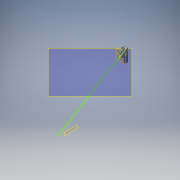
# Autodesk Inventor part: BracerBedMountpoint
Saved by Autodesk Inventor 2016 (Build 200138000, 138)
## iProperties
Created: 2016-05-27
Part Number: BracerBedMountpoint
Material: Generic
Document SubType Name: Modeling
Designer: Scott
Density: 1 g/cm^3
Appearance: Default
Author: Scott
Autodesk Inventor part; units mm, degrees
ref_plane "YZ Plane" through (0, 0, 0) normal (1, 0, 0) x (0, 1, 0)
ref_plane "Work Plane1" through (0, 0, 0) normal (0, 0, 1) x (1, 0, 0)
sketch "Sketch1" plane through (0, 0, 0) normal (0, 0, 1) x (1, 0, 0)
  circle A0 centre (-48.331, 27.8537) radius 2.5 projected
  circle A1 centre (30.6843, -32.9463) radius 2.5 projected
  circle A2 centre (30.6843, -1.1963) radius 2.5 projected
  circle A3 centre (-29.281, 27.8537) radius 2.5 projected
  line L0 (34.412, 17.8537) -> (34.412, 37.8537) projected
  line L1 (34.412, 17.8537) -> (-19.563, 17.8537) projected
  line L2 (-19.563, 37.8537) -> (-19.563, 17.8537) projected
  line L3 (-19.563, 37.8537) -> (-61.031, 37.8537) projected
  line L4 (-61.031, 37.8537) -> (-61.031, 17.8537) projected
  line L5 (-61.031, 17.8537) -> (20.7996, -58.3463) projected
  line L6 (20.7996, -58.3463) -> (40.569, -58.3463) projected
  line L7 (40.569, -58.3463) -> (40.569, 37.8537) projected
  line L8 (40.569, 37.8537) -> (34.412, 37.8537) projected
  line L9 (20.7996, 17.8537) -> (20.7996, -58.3463)
  line L10 (20.7996, 17.8537) -> (34.412, 17.8537)
  line L11 (34.412, 37.8537) -> (34.412, 17.8537)
  point P0 (0, 0)
  constraints: 6 end point, 2 collinear, 1 point on line, 1 vertical
extrude "Extrusion1" add sketch "Sketch1" along normal blind 12.7 contours L0 L8 L7 L6 L9 L1
ref_plane "Work Plane2" through (95.7896, -372.2962, 715.4801) normal (1, 0, 0) x (0, 1, 0)
sketch "Sketch2" plane through (20.7996, 17.8537, 0) normal (0, 1, 0) x (1, 0, 0)
  line L0 (13.6124, 0) -> (-0.6751, -14.2875) projected
  line L1 (13.6124, 0) -> (13.6124, -12.7) projected
  line L2 (13.6124, -12.7) -> (0.9124, -12.7)
  line L3 (13.6124, -12.7) -> (0, -12.7) projected
  line L4 (13.6124, 0) -> (0, 0) projected
  line L5 (13.6124, 0) -> (0.9124, -12.7)
  point P0 (-20.7996, 0)
  constraints: 4 end point, 2 point on line, 1 collinear
extrude "Extrusion2" add sketch "Sketch2" along normal up to surface (20 mm away)
ref_plane "Work Plane3" through (30.569, -58.3463, 0) normal (1, 0, 0) x (0, 0, -1)
sketch "Sketch3" plane through (30.569, -58.3463, 0) normal (1, 0, 0) x (0, 0, -1)
  line L0 (14.0632, 129.5868) -> (-764.5268, -345.4247)
  point P0 (0, 58.3463)
  constraints: 2 end point
ref_plane "Work Plane4" through (30.569, 71.2405, -14.0632) normal (0, -0.5208164, 0.8536687) x (1, 0, 0)
sketch "Sketch4" plane through (30.569, 71.2405, -14.0632) normal (0, -0.5208164, 0.8536687) x (1, 0, 0)
  line L0 (-10, -10) -> (10, -10)
  line L1 (10, -10) -> (10, 10)
  line L2 (10, 10) -> (-10, 10)
  line L3 (-10, 10) -> (-10, -10)
  line L4 (-10, -10) -> (10, 10) construction
  line L5 (10, -10) -> (-10, 10) construction
  point P0 (-30.569, -53.4914)
  point P1 (0, 0)
  dimension "d5" = 20
  dimension "d6" = 20
  constraints: 12 end point, 2 midpoint, 2 parallel, 1 horizontal, 1 perpendicular
  measures "d5" distance of L2.end L1.end
  measures "d6" distance of L1.end L0.end
extrude "Extrusion3" add sketch "Sketch4" along normal blind 76.2
sketch "Sketch5" plane through (40.569, -58.3463, 0) normal (1, 0, 0) x (0, 0, -1)
  line L0 (19.2713, 121.0501) -> (8.855, 138.1235) projected
  line L1 (8.855, 138.1235) -> (-56.1946, 98.4373) projected
  line L2 (-45.7782, 81.3639) -> (-56.1946, 98.4373) projected
  line L3 (19.2713, 121.0501) -> (-45.7782, 81.3639) projected
  line L4 (0, 0) -> (0, 96.2) projected
  line L5 (0, 96.2) -> (-12.7, 96.2) projected
  line L6 (-12.7, 0) -> (-12.7, 96.2) projected
  line L7 (0, 0) -> (-12.7, 0) projected
  line L8 (0, 96.2) -> (26.0499, 96.2)
  line L9 (26.0499, 96.2) -> (26.0499, 148.6139)
  line L10 (26.0499, 148.6139) -> (8.855, 138.1235)
  line L11 (-12.7, 76.2) -> (-12.7, 96.2) projected
  line L12 (-45.7782, 81.3639) -> (-12.7, 76.2)
  point P0 (0, 58.3463)
  constraints: 8 end point, 1 horizontal, 1 perpendicular
extrude "Extrusion4" add sketch "Sketch5" along normal blind 5.08
sketch "Sketch6" plane through (45.649, -58.3463, 0) normal (1, 0, 0) x (0, 0, -1)
  line L0 (0, 0) -> (0, 96.2) projected
  line L1 (0, 96.2) -> (26.0499, 96.2) projected
  line L2 (26.0499, 96.2) -> (26.0499, 148.6139) projected
  line L3 (26.0499, 148.6139) -> (-56.1946, 98.4373) projected
  line L4 (-56.1946, 98.4373) -> (-45.7782, 81.3639) projected
  line L5 (-45.7782, 81.3639) -> (-12.7, 76.2) projected
  line L6 (-12.7, 76.2) -> (-12.7, 0) projected
  line L7 (-12.7, 0) -> (0, 0) projected
  line L8 (0, 0) -> (-12.7, 0) projected
  line L9 (0, 96.2) -> (26.0499, 96.2) projected
  line L10 (-12.7, 0) -> (26.0499, 0)
  line L11 (26.0499, 0) -> (26.0499, 96.2)
  line L12 (26.0499, 96.2) -> (-12.7, 96.2)
  line L13 (-12.7, 96.2) -> (-12.7, 0)
  point P0 (0, 58.3463)
  constraints: 8 end point, 2 parallel, 1 horizontal, 1 perpendicular
extrude "Extrusion5" add sketch "Sketch6" against normal blind 5.08 contours L7 L6 L13 L12 L0 | L0 L1 L11 L10
sketch "Sketch7" plane through (40.569, -58.3463, 0) normal (-1, 0, 0) x (0, 0, 1)
  line L0 (-19.2713, 121.0501) -> (-8.855, 138.1235) projected
  line L1 (12.7, 76.2) -> (12.7, 0) projected
  line L2 (12.7, 0) -> (-26.0499, 0) projected
  line L3 (-26.0499, 0) -> (-26.0499, 148.6139) projected
  line L4 (-26.0499, 148.6139) -> (56.1946, 98.4373) projected
  line L5 (56.1946, 98.4373) -> (45.7782, 81.3639) projected
  line L6 (45.7782, 81.3639) -> (12.7, 76.2) projected
  line L7 (-19.2713, 121.0501) -> (-26.0499, 121.0501)
  line L8 (-26.0499, 148.6139) -> (-26.0499, 0) projected
  line L9 (-8.855, 138.1235) -> (-19.2713, 121.0501) projected
  line L10 (-8.855, 138.1235) -> (-19.2713, 121.0501)
  line L11 (-25.08, 96.2) -> (-5.08, 96.2) projected
  line L12 (-5.08, 96.2) -> (0, 96.2) projected
  line L13 (-19.2713, 121.0501) -> (13.2534, 101.207)
  line L14 (-19.2713, 121.0501) -> (45.7782, 81.3639) projected
  line L15 (0, 96.2) -> (21.4604, 96.2)
  line L16 (0, 96.2) -> (12.7, 96.2) projected
  line L17 (21.4604, 96.2) -> (13.2534, 101.207)
  line L18 (-8.855, 138.1235) -> (-19.2713, 121.0501)
  line L19 (12.7, 76.2) -> (12.7, 96.2) projected
  line L20 (12.7, 96.2) -> (-26.0499, 119.841)
  line L21 (-8.855, 138.1235) -> (-26.0499, 148.6139)
  line L22 (-26.0499, 148.6139) -> (-8.855, 138.1235) projected
  line L23 (-26.0499, 148.6139) -> (-26.0499, 119.841)
  point P0 (0, 58.3463)
  constraints: 18 end point, 7 point on line, 4 collinear, 2 parallel, 1 midpoint, 1 perpendicular
extrude "Extrusion6" add sketch "Sketch7" along normal blind 20 contours L7 L3 L4 L0 | L13 L14 L15 L20 L3 L7 | L14 L6 L19 L15
sketch "Sketch8" plane through (20.569, 61.4947, -26.0499) normal (-1, 0, 0) x (0, 0, 1)
  line L0 (0, 28.7729) -> (82.2445, -21.4037) projected
  line L1 (0, 28.7729) -> (0, 0) projected
  line L2 (0, 0) -> (38.7499, -23.641) projected
  line L3 (38.7499, -23.641) -> (38.7499, -43.641) projected
  line L4 (38.7499, -43.641) -> (71.8281, -38.4771) projected
  line L5 (82.2445, -21.4037) -> (71.8281, -38.4771) projected
  point P0 (26.0499, -61.4947)
extrude "Extrusion7" add sketch "Sketch8" along normal blind 5.08
sketch "Sketch9" plane through (30.569, 31.5543, 50.9864) normal (0, -0.5208164, 0.8536687) x (1, 0, 0)
  line L0 (-15.08, -10) -> (15.08, -10) projected
  line L1 (15.08, 10) -> (15.08, -10) projected
  line L2 (-15.08, 10) -> (15.08, 10) projected
  line L3 (-15.08, -10) -> (-15.08, 10) projected
  line L4 (-15.08, 10) -> (15.08, 10) projected
  line L5 (-15.08, 10) -> (-10, 10)
  line L6 (-10, 10) -> (10, 10)
  line L7 (10, 10) -> (10, -10)
  line L8 (10, -10) -> (-10, -10)
  line L9 (-10, -10) -> (-10, 10)
  point P0 (-30.569, -53.4914)
  dimension "d17" = 5.08
  dimension "d18" = 20
  dimension "d19" = 20
  constraints: 10 end point, 2 parallel, 1 horizontal, 1 perpendicular, 1 point on line
  measures "d17" distance of L2.start L5.end
  measures "d18" distance of L7.end L8.end
  measures "d19" distance of L6.end L7.end
extrude "Extrusion8" cut sketch "Sketch9" against normal blind 73.3425 contours L9 L2 L7 L0
sketch "Sketch10" plane through (40.569, -58.3463, 0) normal (-1, 0, 0) x (0, 0, 1)
  line L0 (12.7, 96.2) -> (-26.0499, 119.841) projected
  line L1 (-26.0499, 119.841) -> (-26.0499, 0) projected
  line L2 (-26.0499, 0) -> (0, 0) projected
  line L3 (0, 96.2) -> (0, 0) projected
  line L4 (0, 96.2) -> (12.7, 96.2) projected
  line L5 (12.7, 96.2) -> (0, 96.2) projected
  line L6 (0, 96.2) -> (-26.0499, 96.2)
  line L7 (-26.0499, 0) -> (-26.0499, 148.6139) projected
  line L8 (-26.0499, 96.2) -> (-26.0499, 101.28)
  line L9 (-26.0499, 101.28) -> (4.3734, 101.28)
  line L10 (12.7, 96.2) -> (-26.0499, 119.841) projected
  line L11 (4.3734, 101.28) -> (12.7, 96.2)
  line L12 (-26.0499, 101.28) -> (-6.0499, 101.28)
  line L13 (-6.0499, 101.28) -> (-6.0499, 96.2)
  line L14 (-6.0499, 96.2) -> (-26.0499, 96.2)
  line L15 (-26.0499, 96.2) -> (-26.0499, 101.28)
  point P0 (0, 58.3463)
  dimension "d22" = 5.08
  dimension "d23" = 20
  constraints: 16 end point, 6 point on line, 2 collinear, 2 parallel, 2 perpendicular, 1 horizontal
  measures "d22" distance of L6.end L8.end
  measures "d23" distance of L13.end L14.end
extrude "Extrusion9" add sketch "Sketch10" along normal blind 76.2 contours L13 L6 L1 L9
sketch "Sketch11" plane through (15.489, 61.4947, -26.0499) normal (-1, 0, 0) x (0, 0, 1)
  line L0 (0, 0) -> (0, -18.561)
  line L1 (0, -18.561) -> (20, -18.561)
  line L2 (20, -18.561) -> (40.523, -19.3781)
  line L3 (71.8281, -38.4771) -> (9.2179, -0.2791) projected
  line L4 (0, 0) -> (38.7499, -23.641) projected
  line L5 (0, 0) -> (40.523, -19.3781)
  point P0 (26.0499, -61.4947)
  constraints: 8 end point, 1 midpoint, 1 perpendicular, 1 vertical
extrude "Extrusion10" add sketch "Sketch11" against normal blind 5.08
sketch "Sketch12" plane through (15.489, 61.4947, -26.0499) normal (-1, 0, 0) x (0, 0, 1)
  line L0 (82.2445, -21.4037) -> (71.8281, -38.4771) projected
  line L1 (19.6343, 16.7942) -> (82.2445, -21.4037) projected
  line L2 (19.6343, 16.7942) -> (9.2179, -0.2791) projected
  line L3 (71.8281, -38.4771) -> (9.2179, -0.2791) projected
  circle A0 centre (63.0438, -21.4037) radius 2.5
  circle A1 centre (34.4445, -3.9555) radius 2.5
  point P0 (26.0499, -61.4947)
  dimension "d28" = 5
  dimension "d29" = 5
  constraints: 2 centre point
  measures "d28" diameter of A0
  measures "d29" diameter of A1
extrude "Extrusion11" cut sketch "Sketch12" against normal blind 76.2 contours A0 | A1
sketch "Sketch13" plane through (21.712, 17.8537, 12.7) normal (0, -0.9880329, 0.154243) x (1, 0, 0)
  point P0 (-21.712, -15.3018)
ref_plane "Work Plane5" through (-12.4192, 17.8537, 7.1437) normal (0, -1, 0) x (0.7071068, 0, 0.7071068)
ref_plane "Work Plane6" through (-5.2755, 17.8537, 0) normal (0, -1, 0) x (1, 0, 0)
sketch "Sketch14" plane through (-5.2755, 17.8537, 0) normal (0, -1, 0) x (1, 0, 0)
  circle A0 centre (13.1445, 17.7848) radius 4 projected
  line L0 (46.2678, -5.1058) -> (-55.3321, -5.0122) projected
  line L1 (46.2678, -5.1058) -> (46.2725, -0.0258) projected
  line L2 (46.2725, -0.0258) -> (40.1156, -0.0201) projected
  line L3 (40.1156, -0.0201) -> (25.8412, 14.2805) projected
  line L4 (25.8412, 14.2805) -> (25.8515, 25.393) projected
  line L5 (25.8515, 25.393) -> (0.4515, 25.4165) projected
  line L6 (0.4412, 14.304) -> (0.4515, 25.4165) projected
  line L7 (0.4412, 14.304) -> (-13.8594, 0.0296) projected
  line L8 (-13.8594, 0.0296) -> (-55.3275, 0.0678) projected
  line L9 (-55.3321, -5.0122) -> (-55.3275, 0.0678) projected
  line L10 (20.7645, 56.1946) -> (20.7645, -26.0499) projected
  line L11 (20.7645, 25.3977) -> (20.7645, 11.9655)
  line L12 (27.7015, 12.4168) -> (20.7645, 12.4168)
  point P0 (5.2755, 0)
  constraints: 5 point on line, 4 end point, 1 perpendicular
ref_plane "Work Plane7" through (-61.031, 37.8537, -5.08) normal (0, 1, 0) x (0, 0, 1)
extrude "Extrusion12" cut sketch "Sketch14" against normal up to surface (20 mm away) contours L10 L5 L4 L3 L12
sketch "Sketch15" plane through (45.649, -58.3463, 0) normal (1, 0, 0) x (0, 0, -1)
  line L0 (-45.7782, 81.3639) -> (16.832, 119.5619) projected
  line L1 (-12.7, 54.65) -> (-12.7, 59.65) projected
  line L2 (-45.7782, 81.3639) -> (-12.7, 59.65)
  line L3 (-12.7, 76.2) -> (-12.7, 0) projected
  line L4 (-12.7, 59.65) -> (-12.7, 76.2)
  line L5 (-12.7, 76.2) -> (-45.7782, 81.3639)
  line L6 (-25.393, 78.1815) -> (-14.2805, 76.4467) projected
  point P0 (0, 58.3463)
  constraints: 6 end point, 2 collinear
extrude "Extrusion13" add sketch "Sketch15" against normal blind 2.54
sketch "Sketch16" plane through (15.489, 61.4947, -26.0499) normal (-1, 0, 0) x (0, 0, 1)
  line L0 (38.7499, -60.191) -> (71.8281, -38.4771) projected
  line L1 (38.7499, -43.641) -> (71.8281, -38.4771) projected
  line L2 (38.7499, -60.191) -> (38.7499, -43.641) projected
  point P0 (26.0499, -61.4947)
sketch "Sketch17" plane through (20.7996, -58.3463, 0) normal (0, -1, 0) x (1, 0, 0)
  line L0 (-0.2306, 45.7782) -> (-0.2306, 56.1946) projected
  line L1 (-0.2306, 56.1946) -> (-0.2306, 26.8017)
  line L2 (-0.2306, 56.1946) -> (-0.2306, -6.4156) projected
  line L3 (-0.2306, 26.8017) -> (-35.0854, 26.8017)
  line L4 (-35.0854, 26.8017) -> (-32.5569, 61.6946)
  line L5 (-32.5569, 61.6946) -> (-0.2306, 56.1946)
  point P0 (-20.7996, 0)
  constraints: 8 end point, 1 horizontal, 1 point on line
extrude "Extrusion14" cut sketch "Sketch17" against normal blind 508
sketch "Sketch18" plane through (45.649, -58.3463, -26.0499) normal (0, 0, -1) x (-1, 0, 0)
  line L0 (30.16, 148.6139) -> (30.16, 101.28) projected
  line L1 (30.16, 101.28) -> (81.28, 101.28) projected
  line L2 (30.16, 148.6139) -> (81.28, 101.28)
  line L3 (81.28, 101.28) -> (30.16, 101.28)
  line L4 (30.16, 78.4014) -> (30.16, 116.3696) projected
  line L5 (30.16, 101.28) -> (30.16, 148.6139)
  point P0 (45.649, 58.3463)
  constraints: 6 end point, 2 perpendicular
extrude "Extrusion15" add sketch "Sketch18" against normal blind 2.54
sketch "Sketch19" plane through (-35.631, 42.9337, -6.0499) normal (0, 1, 0) x (1, 0, 0)
  line L0 (0, 0) -> (0, 17.46) projected
  line L1 (51.12, 0) -> (0, 0) projected
  line L2 (0, 20) -> (51.12, 20) projected
  line L3 (0, 20) -> (0, 0) projected
  line L4 (0, 0) -> (0, 20)
  line L5 (0, 10) -> (12.7, 10)
  circle A0 centre (12.7, 10) radius 2.5
  line L6 (12.7, 10) -> (38.1, 10)
  line L7 (51.12, -32.8516) -> (51.12, 17.46) projected
  line L8 (12.7, 10) -> (38.1, 10) construction
  circle A1 centre (38.1, 10) radius 2.5
  point P0 (35.631, -6.0499)
  dimension "d40" = 12.7
  dimension "d41" = 5
  dimension "d42" = 25.4
  dimension "d43" = 0
  dimension "d44" = 5
  constraints: 8 end point, 2 centre point, 2 coincident, 2 collinear, 2 horizontal, 1 midpoint, 1 perpendicular
  measures "d40" distance of L5.start L5.end
  measures "d41" diameter of A0
  measures "d42" distance of L6.start L6.end
  measures "d43" distance between parallel lines of L6 L8
  measures "d44" diameter of A1
extrude "Extrusion16" cut sketch "Sketch19" against normal blind 32.385
sketch "Sketch20" plane through (45.649, -58.3463, 0) normal (1, 0, 0) x (0, 0, -1)
  line L0 (5.08, 76.2) -> (5.08, -800.1) projected
  line L1 (25.08, -800.1) -> (5.08, -800.1) projected
  line L2 (25.08, 76.2) -> (25.08, -800.1) projected
  line L3 (5.08, 76.2) -> (25.08, 76.2) projected
  circle A0 centre (15.08, 12.1289) radius 2.5
  circle A1 centre (15.08, 48.2566) radius 2.5
  point P0 (0, 58.3463)
  dimension "d47" = 5
  dimension "d48" = 5
  constraints: 2 centre point
  measures "d47" diameter of A0
  measures "d48" diameter of A1
extrude "Extrusion17" cut sketch "Sketch20" against normal blind 32.385 contours A0 | A1
sketch "Sketch21" plane through (45.649, -58.3463, 0) normal (1, 0, 0) x (0, 0, -1)
  line L0 (5.08, 76.2) -> (5.08, -800.1) projected
  line L1 (25.08, -800.1) -> (5.08, -800.1) projected
  line L2 (25.08, 76.2) -> (25.08, -800.1) projected
  line L3 (5.08, 76.2) -> (25.08, 76.2) projected
  circle A0 centre (15.08, 12.1289) radius 2.5 projected
  circle A1 centre (15.08, 48.2566) radius 2.5 projected
  circle A2 centre (-36.9939, 98.4373) radius 2.5 projected
  circle A3 centre (-8.3946, 115.8855) radius 2.5 projected
  line L4 (-12.7, 59.65) -> (-12.7, 0) projected
  line L5 (-12.7, 0) -> (26.0499, 0) projected
  line L6 (26.0499, 0) -> (26.0499, 148.6139) projected
  line L7 (26.0499, 148.6139) -> (-56.1946, 98.4373) projected
  line L8 (-56.1946, 98.4373) -> (-45.7782, 81.3639) projected
  line L9 (-45.7782, 81.3639) -> (-12.7, 59.65) projected
  line L10 (-12.7, 59.65) -> (-8.3946, 56.8238)
  line L11 (-8.3946, 56.8238) -> (-8.3946, 0)
  line L12 (-12.7, 0) -> (26.0499, 0) projected
  point P0 (0, 58.3463)
  constraints: 4 end point, 1 perpendicular, 1 point on line
extrude "Extrusion18" cut sketch "Sketch21" against normal blind 54.9275 contours L5 L4 L10 L11
sketch "Sketch22" plane through (45.649, -58.3463, 8.3946) normal (0, 0, 1) x (1, 0, 0)
  arc A0 (-17.4433, 56.8238) -> (-12.4861, 56.8238) centre (-14.9647, 57.15) ccw projected
  circle A1 centre (-14.9647, 57.15) radius 5.08
  point P0 (-45.649, 58.3463)
  dimension "d53" = 10.16
  constraints: 1 centre point, 1 coincident
  measures "d53" diameter of A1
extrude "Extrusion19" cut sketch "Sketch22" along normal blind 43.4975
sketch "Sketch23" plane through (30.569, 31.5543, 50.9864) normal (0, -0.5208164, 0.8536687) x (1, 0, 0)
  line L0 (10, -10) -> (10, 10) projected
  line L1 (10, 10) -> (-10, 10) projected
  line L2 (-10, 10) -> (-10, -10) projected
  line L3 (-10, -10) -> (10, -10) projected
  line L4 (-15.08, 10) -> (15.08, 10) projected
  line L5 (10.5, -10) -> (-10.5, -10)
  line L6 (-10.5, -10) -> (-10.5, 10)
  line L7 (-10.5, 10) -> (10.5, 10)
  line L8 (10.5, 10) -> (10.5, -10)
  line L9 (10.5, -10) -> (-10.5, 10) construction
  line L10 (-10.5, -10) -> (10.5, 10) construction
  point P0 (-30.569, -53.4914)
  point P1 (0, 0)
  dimension "d56" = 21
  constraints: 12 end point, 2 midpoint, 2 parallel, 1 horizontal, 1 perpendicular, 1 point on line
  measures "d56" distance of L6.end L7.end
ref_plane "Work Plane8" through (19.569, 60.3619, -17.3528) normal (0, -0.5208164, 0.8536687) x (1, 0, 0)
extrude "Extrusion20" cut sketch "Sketch23" against normal up to surface (73.3425 mm away) contours L3 L2 L1 L0
body "Solid1"
